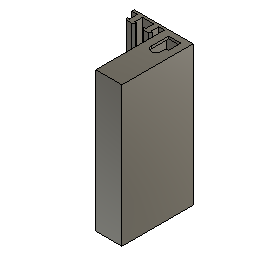
Battery Holder v1 (Autodesk Fusion 360 design; units mm, degrees)
Autodesk Fusion 360 part; units mm, degrees
sketch "Sketch1" plane through (0, 0, 0) normal (0, 0, 1) x (1, 0, 0)
  line L0 (0, 0) -> (6.9, 0)
  line L1 (6.9, 0) -> (6.9, -9.4)
  line L2 (6.9, -9.4) -> (4.6, -9.4)
  line L3 (4.6, -9.4) -> (4.6, -10.4)
  line L4 (4.6, -10.4) -> (6.9335, -12.7335)
  line L5 (4.6, -10.4) -> (7.9, -10.4) construction
  line L6 (4.6, -9.4) -> (10.8, -9.4)
  line L7 (6.9, -9.4) -> (13.1, -9.4)
  line L8 (13.1, -9.4) -> (15.4, -9.4)
  line L9 (15.4, -9.4) -> (15.4, -10.4)
  line L10 (15.4, -10.4) -> (13.0665, -12.7335)
  line L11 (13.0665, -12.7335) -> (6.9335, -12.7335)
  line L12 (15.4, -9.4) -> (13.1, -9.4)
  line L13 (13.1, -9.4) -> (13.1, 0)
  line L14 (13.1, 0) -> (20.1, 0)
  line L15 (20.1, 0) -> (20.1, 3)
  line L16 (20.1, 3) -> (0, 3)
  line L17 (0, 3) -> (0, 0)
  dimension "d1" = 6.9
  dimension "d2" = 9.4
  dimension "d3" = 2.3
  dimension "d4" = 1
  dimension "d5" = 45
  dimension "d6" = 3.3
  dimension "d7" = 6.2
  dimension "d11" = 6.2
  dimension "d12" = 135
  dimension "d13" = 3.3
  dimension "d14" = 7
  dimension "d118" = 2.3
  dimension "d119" = 9.4
  dimension "d120" = 3
  constraint coincident L0.start L17.end
  constraint horizontal L0
  constraint perpendicular L0 L1
  constraint perpendicular L1 L2
  constraint perpendicular L2 L3
  constraint horizontal L5
  constraint perpendicular L3 L6
  constraint perpendicular L1 L7
  constraint parallel L7 L8
  constraint perpendicular L8 L9
  constraint perpendicular L12 L13
  constraint perpendicular L13 L14
  constraint perpendicular L14 L15
  constraint perpendicular L15 L16
  constraint perpendicular L0 L17
  constraint parallel L6 L11
  measures "d1" distance of L0.start L0.end
  measures "d2" distance of L0.end L1.end
  measures "d3" distance of L1.end L2.end
  measures "d4" distance of L2.end L3.end
  measures "d5" angle of L4 L5
  measures "d6" distance of L3.end L4.end
  measures "d7" distance of L2.end L6.end
  measures "d11" distance of L1.end L7.end
  measures "d12" angle of L9 L10
  measures "d13" distance of L9.end L10.end
  measures "d14" distance of L13.end L14.end
  measures "d118" distance of L7.end L8.end
  measures "d119" distance of L7.end L13.end
  measures "d120" distance of L14.end L15.end
extrude "Extrude1" add sketch "Sketch1" along normal blind 171
mirror "Mirror1" about plane through (0, 0, 0) normal (1, 0, 0) of bodies 1 merged
sketch "Sketch10" plane through (20.1, 0, 0) normal (1, 0, 0) x (0, 1, 0)
  line L0 (0, 0) -> (3, 0)
  line L1 (3, 0) -> (3, 171)
  line L2 (3, 171) -> (0, 171)
  line L3 (0, 171) -> (0, 0)
  line L4 (3, 171) -> (3, 0)
  line L5 (3, 0) -> (-84, 0)
  line L6 (-84, 0) -> (-84, 171)
  line L7 (-84, 171) -> (3, 171)
  dimension "d121" = 171
  dimension "d122" = 87
  constraint perpendicular L4 L5
  constraint parallel L4 L6
  constraint parallel L5 L7
  constraint perpendicular L2 L4
  constraint coincident L1.end L2.start
  measures "d121" distance of L1.end L0.end
  measures "d122" distance of L1.end L6.end
extrude "Extrude33" add sketch "Sketch10" along normal blind 32
sketch "Sketch11" plane through (0, 0, 0) normal (0, 0, -1) x (1, 0, 0)
  line L0 (13.1, 9.4) -> (15.4, 9.4)
  line L1 (15.4, 9.4) -> (15.4, 10.4)
  line L2 (15.4, 10.4) -> (13.0665, 12.7335)
  line L3 (13.0665, 12.7335) -> (6.9335, 12.7335)
  line L4 (6.9335, 12.7335) -> (4.6, 10.4)
  line L5 (4.6, 10.4) -> (4.6, 9.4)
  line L6 (4.6, 9.4) -> (6.9, 9.4)
  line L7 (6.9, 9.4) -> (6.9, 0)
  line L8 (6.9, 0) -> (-6.9, 0)
  line L9 (-6.9, 0) -> (-6.9, 9.4)
  line L10 (-6.9, 9.4) -> (-4.6, 9.4)
  line L11 (-4.6, 9.4) -> (-4.6, 10.4)
  line L12 (-4.6, 10.4) -> (-6.9335, 12.7335)
  line L13 (-6.9335, 12.7335) -> (-13.0665, 12.7335)
  line L14 (-13.0665, 12.7335) -> (-15.4, 10.4)
  line L15 (-15.4, 10.4) -> (-15.4, 9.4)
  line L16 (-15.4, 9.4) -> (-13.1, 9.4)
  line L17 (-13.1, 9.4) -> (-13.1, 0)
  line L18 (-13.1, 0) -> (-20.1, 0)
  line L19 (-20.1, 0) -> (-20.1, -3)
  line L20 (-20.1, -3) -> (52.1, -3)
  line L21 (52.1, -3) -> (52.1, 84)
  line L22 (52.1, 84) -> (20.1, 84)
  line L23 (20.1, 84) -> (20.1, 0)
  line L24 (20.1, 0) -> (13.1, 0)
  line L25 (13.1, 0) -> (13.1, 9.4)
  line L26 (49.1, 0) -> (23.1, 0)
  line L27 (23.1, 0) -> (23.1, 81)
  line L28 (23.1, 81) -> (49.1, 81)
  line L29 (49.1, 81) -> (49.1, 0)
  line L30 (49.1, 0) -> (23.1, 81) construction
  line L31 (23.1, 0) -> (49.1, 81) construction
  point P0 (36.1, 40.5)
  dimension "d127" = 3
  dimension "d128" = 3
  dimension "d130" = 3
  dimension "d131" = 3
  constraint horizontal L26
  constraint perpendicular L26 L27
  constraint parallel L26 L28
  constraint parallel L27 L29
  constraint coincident L30 P0
  constraint coincident L31 P0
  measures "d127" distance of L23 L27
  measures "d128" distance of L21 L29
  measures "d130" distance of L22 L28
  measures "d131" distance of L20 L26
extrude "Extrude34" cut sketch "Sketch11" against normal blind 168 contours L26 L27 L28 L29
sketch "Sketch12" plane through (20.1, 0, 0) normal (-1, 0, 0) x (0, -1, 0)
  line L0 (0, 171) -> (0, 0)
  line L1 (0, 0) -> (84, 0)
  line L2 (84, 0) -> (84, 171)
  line L3 (84, 171) -> (0, 171)
  line L4 (39, 40) -> (17.1845, 40)
  line L5 (17.1845, 40) -> (17.1845, 131)
  line L6 (17.1845, 131) -> (39, 131)
  line L7 (39, 131) -> (39, 40)
  dimension "d134" = 45
  dimension "d135" = 40
  dimension "d136" = 40
  constraint horizontal L4
  constraint vertical L5
  constraint horizontal L6
  constraint vertical L7
  measures "d134" distance of L2 L7
  measures "d135" distance of L1 L4
  measures "d136" distance of L3 L6
extrude "Extrude35" cut sketch "Sketch12" against normal blind 3 contours L4 L5 L6 L7
sketch "Sketch13" plane through (0, 0, 0) normal (0, 0, -1) x (1, 0, 0)
  line L0 (23.1, 0) -> (23.1, 81)
  line L1 (23.1, 81) -> (49.1, 81)
  line L2 (49.1, 81) -> (49.1, 0)
  line L3 (49.1, 0) -> (23.1, 0)
  line L4 (13.1, 9.4) -> (15.4, 9.4)
  line L5 (15.4, 9.4) -> (15.4, 10.4)
  line L6 (15.4, 10.4) -> (13.0665, 12.7335)
  line L7 (13.0665, 12.7335) -> (6.9335, 12.7335)
  line L8 (6.9335, 12.7335) -> (4.6, 10.4)
  line L9 (4.6, 10.4) -> (4.6, 9.4)
  line L10 (4.6, 9.4) -> (6.9, 9.4)
  line L11 (6.9, 9.4) -> (6.9, 0)
  line L12 (6.9, 0) -> (-6.9, 0)
  line L13 (-6.9, 0) -> (-6.9, 9.4)
  line L14 (-6.9, 9.4) -> (-4.6, 9.4)
  line L15 (-4.6, 9.4) -> (-4.6, 10.4)
  line L16 (-4.6, 10.4) -> (-6.9335, 12.7335)
  line L17 (-6.9335, 12.7335) -> (-13.0665, 12.7335)
  line L18 (-13.0665, 12.7335) -> (-15.4, 10.4)
  line L19 (-15.4, 10.4) -> (-15.4, 9.4)
  line L20 (-15.4, 9.4) -> (-13.1, 9.4)
  line L21 (-13.1, 9.4) -> (-13.1, 0)
  line L22 (-13.1, 0) -> (-20.1, 0)
  line L23 (-20.1, 0) -> (-20.1, -3)
  line L24 (-20.1, -3) -> (52.1, -3)
  line L25 (52.1, -3) -> (52.1, 84)
  line L26 (52.1, 84) -> (20.1, 84)
  line L27 (20.1, 84) -> (20.1, 0)
  line L28 (20.1, 0) -> (13.1, 0)
  line L29 (13.1, 0) -> (13.1, 9.4)
  line L30 (52.1, 84) -> (20.1, 84)
  line L31 (20.1, 84) -> (20.1, 59)
  line L32 (20.1, 59) -> (52.1, 59)
  line L33 (52.1, 59) -> (52.1, 84)
  dimension "d139" = 25
  constraint horizontal L30
  constraint vertical L31
  constraint horizontal L32
  constraint vertical L33
  constraint coincident L25.end L26.start
  measures "d139" distance of L25.end L32.end
extrude "Extrude36" add sketch "Sketch13" against normal blind 3 contours L0 L1 L2 L25 L26 L27 L30 L31 L32 L33 | L0 L1 L2 L32
sketch "Sketch14" plane through (0, 0, 171) normal (0, 0, 1) x (-1, 0, 0)
  line L0 (-15.4, 9.4) -> (-13.1, 9.4)
  line L1 (-13.1, 9.4) -> (-13.1, 0)
  line L2 (-13.1, 0) -> (-20.1, 0)
  line L3 (-20.1, 0) -> (-20.1, 84)
  line L4 (-20.1, 84) -> (-52.1, 84)
  line L5 (-52.1, 84) -> (-52.1, -3)
  line L6 (-52.1, -3) -> (20.1, -3)
  line L7 (20.1, -3) -> (20.1, 0)
  line L8 (20.1, 0) -> (13.1, 0)
  line L9 (13.1, 0) -> (13.1, 9.4)
  line L10 (13.1, 9.4) -> (15.4, 9.4)
  line L11 (15.4, 9.4) -> (15.4, 10.4)
  line L12 (15.4, 10.4) -> (13.0665, 12.7335)
  line L13 (13.0665, 12.7335) -> (6.9335, 12.7335)
  line L14 (6.9335, 12.7335) -> (4.6, 10.4)
  line L15 (4.6, 10.4) -> (4.6, 9.4)
  line L16 (4.6, 9.4) -> (6.9, 9.4)
  line L17 (6.9, 9.4) -> (6.9, 0)
  line L18 (6.9, 0) -> (-6.9, 0)
  line L19 (-6.9, 0) -> (-6.9, 9.4)
  line L20 (-6.9, 9.4) -> (-4.6, 9.4)
  line L21 (-4.6, 9.4) -> (-4.6, 10.4)
  line L22 (-4.6, 10.4) -> (-6.9335, 12.7335)
  line L23 (-6.9335, 12.7335) -> (-13.0665, 12.7335)
  line L24 (-13.0665, 12.7335) -> (-15.4, 10.4)
  line L25 (-15.4, 10.4) -> (-15.4, 9.4)
  line L26 (-28.9884, 3.794) -> (-43.9884, 3.794)
  line L27 (-43.9884, 3.794) -> (-43.9884, 18.794)
  line L28 (-43.9884, 18.794) -> (-28.9884, 18.794)
  line L29 (-28.9884, 18.794) -> (-28.9884, 3.794)
  line L30 (-28.9884, 18.794) -> (-28.9884, 30.794)
  line L31 (-28.9884, 30.794) -> (-40.9884, 30.794)
  line L32 (-40.9884, 30.794) -> (-40.9884, 18.794)
  dimension "d142" = 15
  dimension "d143" = 15
  dimension "d148" = 12
  dimension "d149" = 12
  constraint horizontal L26
  constraint vertical L27
  constraint horizontal L28
  constraint vertical L29
  constraint perpendicular L28 L30
  constraint perpendicular L29 L31
  constraint coincident L28 L32.end
  constraint perpendicular L28 L32
  measures "d142" distance of L26.start L26.end
  measures "d143" distance of L26.start L28.end
  measures "d148" distance of L28.end L30.end
  measures "d149" distance of L30.end L31.end
extrude "Extrude37" cut sketch "Sketch14" against normal blind 3 contours L26 L27 L28 L29 | L28 L30 L31 L32
fillet "Fillet5" radius 6 1 edges at (40.9884, -30.794, 169.5)
fillet "Fillet6" radius 6 1 edges at (28.9884, -30.794, 169.5)
